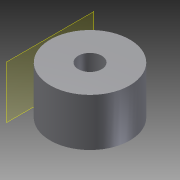
# Autodesk Inventor part: OCT_Adapter_Bottom
Saved by Autodesk Inventor 2011 SP2 (Build 150309200, 309)
## iProperties
Created: 2012-03-27
Part Number: OCT_Adapter_Bottom
Document SubType Name: Modeling
Designer: sungwook
Density: 1 g/cm^3
Author: sungwook
Autodesk Inventor part; units mm, degrees
ref_plane "XZ Plane" through (0, 0, 0) normal (0, 1, 0) x (-1, 0, 0)
ref_plane "XY Plane" through (0, 0, 0) normal (0, 0, 1) x (1, 0, 0)
sketch "Sketch1" plane through (0, 0, 0) normal (0, 0, 1) x (1, 0, 0)
  circle A0 centre (0, 0) radius 2.5
  dimension "d0" = 5
  constraints: 1 centre point, 1 coincident
  measures "d0" diameter of A0
extrude "Extrusion1" add sketch "Sketch1" along normal blind 3
hole "Hole1" at (0, 0, 3) direction (0, 0, -1) diameter 1.4732 end through all
ref_plane "Work Plane1" through (-2.5, 0, 0) normal (1, 0, 0) x (0, 1, 0)
sketch "Sketch2" plane through (-2.5, 0, 0) normal (1, 0, 0) x (0, 1, 0)
  line L0 (-2.5, 3) -> (2.5, 3) projected
  line L1 (-2.5, 0) -> (2.5, 0) projected
  line L2 (0, -0.6) -> (0, 3.6) projected
  point P0 (0, 0)
  point P1 (0, 1.5)
  dimension "d12" = 1.5
  constraints: 1 midpoint
  measures "d12" distance of point (0, 1.5) point (0, 0)
hole "Hole2" at (-2.5, 0, 1.5) direction (1, 0, 0) diameter 1.181 depth 2.5 thread size "0-80 UNF" class "2B" standard "ANSI Unified Screw Threads"
body "Solid1"
